script OS 6_v1 (Autodesk Fusion 360 design; units mm, degrees)
Autodesk Fusion 360 part; units mm, degrees
(part 1 of 3)
sketch "right content" plane through (0, 0, 0) normal (0, 0, 1) x (1, 0, 0)
  line L0 (-306, -8) -> (-256, -8) construction
  line L1 (-256, -128) -> (-306, -128) construction
  line L2 (-256, -8) -> (-256, -128) construction
  line L3 (-306, -128) -> (-306, -8) construction
  circle A0 centre (-298, -98) radius 1.005 construction
  point P0 (-294, -98)
  point P1 (-290, -98)
  point P2 (-298, -94)
  point P3 (-294, -94)
  point P4 (-290, -94)
  point P5 (-298, -90)
  point P6 (-294, -90)
  point P7 (-290, -90)
  point P8 (-298, -86)
  point P9 (-294, -86)
  point P10 (-290, -86)
  point P11 (-298, -82)
  point P12 (-294, -82)
  point P13 (-290, -82)
  point P14 (-298, -78)
  point P15 (-294, -78)
  point P16 (-290, -78)
  point P17 (-298, -74)
  point P18 (-294, -74)
  point P19 (-290, -74)
  point P20 (-298, -70)
  point P21 (-294, -70)
  point P22 (-290, -70)
  point P23 (-298, -66)
  point P24 (-294, -66)
  point P25 (-290, -66)
  point P26 (-298, -62)
  point P27 (-294, -62)
  point P28 (-290, -62)
  dimension "d85" = 50
  dimension "d390" = 120
  dimension "d391" = 2.01
  dimension "d394" = 4
  dimension "d395" = 4
  dimension "d403" = 30
  dimension "d404" = 8
  constraint horizontal L1
  constraint horizontal L0
  constraint vertical L2
  constraint vertical L3
  constraint coincident L1.end L3.start
  constraint coincident L0.end L2.start
  measures "d85" distance of L0.start L0.end
  measures "d390" distance of L0 L1
  measures "d391" diameter of A0
  measures "d403" distance of L1 A0.centre
  measures "d404" distance of L3 A0.centre
sketch "top content" plane through (0, 0, 0) normal (0, 0, 1) x (1, 0, 0)
  circle A0 centre (75, 95) radius 6.5
  circle A1 centre (20, 25) radius 6.5
  circle A2 centre (90.5, 79.5) radius 1.588
  circle A3 centre (59.5, 79.5) radius 1.588
  circle A4 centre (90.5, 110.5) radius 1.588
  circle A5 centre (59.5, 110.5) radius 1.588
  circle A6 centre (130, 25) radius 6.5
  line L0 (0, 0) -> (0, 120) construction
  line L1 (0, 120) -> (150, 120) construction
  line L2 (150, 120) -> (150, 0) construction
  line L3 (150, 0) -> (0, 0) construction
  line L4 (0, 0) -> (150, 120) construction
  line L5 (0, 120) -> (150, 0) construction
  line L6 (75, 0) -> (75, 120) construction
  point P0 (75, 60)
  dimension "d263" = 31
  dimension "d25" = 31
  dimension "d3" = 13
  dimension "d4" = 110
  dimension "d272" = 3.176
  dimension "d1371" = 120
  dimension "d1372" = 150
  dimension "d1373" = 25
  dimension "d1374" = 25
  dimension "d2151" = 15.5
  dimension "d2152" = 15.5
  dimension "d2153" = 55
  dimension "d2154" = 35
  constraint equal A0 A1
  constraint equal A1 A6
  constraint perpendicular L0 L1
  constraint parallel L0 L2
  constraint parallel L1 L3
  constraint coincident L4 P0
  constraint coincident L5 P0
  constraint midpoint L3 L6.start
  constraint midpoint L1 L6.end
  constraint coincident A0.centre L6
  constraint horizontal L3
  measures "d3" diameter of A1
  measures "d4" distance of A6.centre A1.centre
  measures "d272" diameter of A3
  measures "d1371" distance of L1.end L2.end
  measures "d1372" distance of L0.end L1.end
  measures "d1373" distance of A0.centre L1
  measures "d1374" distance of A6.centre L3
  measures "d2151" horizontal distance of A0.centre A2.centre
  measures "d2152" vertical distance of A0.centre A4.centre
  measures "d2153" horizontal distance of A1.centre P0
  measures "d2154" vertical distance of A1.centre P0
sketch "bottom content" plane through (0, 0, 0) normal (0, 0, 1) x (1, 0, 0)
  circle A0 centre (245.4709, 45.6033) radius 1
  circle A1 centre (385.4709, 45.6033) radius 1
  circle A2 centre (245.4709, -54.3967) radius 1
  circle A3 centre (385.4709, -54.3967) radius 1
  circle A4 centre (255.4709, 35.6033) radius 1
  circle A5 centre (375.4709, 35.6033) radius 1
  circle A6 centre (255.4709, -44.3967) radius 1
  circle A7 centre (375.4709, -44.3967) radius 1
  line L0 (235.4709, 55.6033) -> (395.4709, 55.6033) construction
  line L1 (395.4709, 55.6033) -> (395.4709, -64.3967) construction
  line L2 (395.4709, -64.3967) -> (235.4709, -64.3967) construction
  line L3 (235.4709, -64.3967) -> (235.4709, 55.6033) construction
  line L4 (235.4709, 55.6033) -> (395.4709, -64.3967) construction
  line L5 (395.4709, 55.6033) -> (235.4709, -64.3967) construction
  line L6 (268.4709, -6.3967) -> (362.4709, -6.3967) construction
  line L7 (362.4709, -6.3967) -> (362.4709, -54.3967) construction
  line L8 (362.4709, -54.3967) -> (268.4709, -54.3967) construction
  line L9 (268.4709, -54.3967) -> (268.4709, -6.3967) construction
  line L10 (315.4709, -4.3967) -> (315.4709, -64.3967) construction
  circle A8 centre (268.4709, -6.3967) radius 1
  circle A9 centre (362.4709, -6.3967) radius 1
  circle A10 centre (362.4709, -54.3967) radius 1
  circle A11 centre (268.4709, -54.3967) radius 1
  point P0 (315.4709, -4.3967)
  point P1 (315.4709, -4.3967)
  dimension "d282" = 2
  dimension "d287" = 140
  dimension "d288" = -100
  dimension "d289" = 2
  dimension "d294" = 120
  dimension "d295" = -80
  dimension "d356" = 160
  dimension "d357" = 120
  dimension "d358" = 70
  dimension "d359" = 50
  dimension "d360" = 60
  dimension "d361" = 40
  dimension "d362" = 94
  dimension "d363" = 48
  dimension "d364" = 10
  dimension "d365" = 47
  dimension "d366" = 2
  dimension "d368" = 2
  dimension "d369" = 2
  dimension "d370" = 2
  constraint horizontal L0
  constraint perpendicular L0 L1
  constraint parallel L0 L2
  constraint parallel L1 L3
  constraint coincident L4 P1
  constraint coincident L5 P1
  constraint coincident P1 P0
  constraint horizontal L6
  constraint vertical L7
  constraint horizontal L8
  constraint vertical L9
  constraint midpoint L2 L10.end
  constraint coincident L6.start L9.end
  constraint coincident L6.end L7.start
  constraint coincident L7.end L8.start
  constraint coincident L8.end L9.start
  measures "d282" diameter of A0
  measures "d289" diameter of A4
  measures "d356" distance of L1.end L2.end
  measures "d357" distance of L0.start L2.end
  measures "d358" horizontal distance of A0.centre P0
  measures "d359" vertical distance of A0.centre P0
  measures "d360" horizontal distance of A4.centre P1
  measures "d361" vertical distance of A4.centre P1
  measures "d362" distance of L6.start L6.end
  measures "d363" distance of L6.start L8.end
  measures "d364" distance of L2 L8
  measures "d365" distance of L8.end L10
  measures "d366" diameter of A8
  measures "d368" diameter of A11
  measures "d369" diameter of A9
  measures "d370" diameter of A10
sketch "back content" plane through (0, 0, 0) normal (0, 0, 1) x (1, 0, 0)
  line L0 (16.9082, 180.3872) -> (176.9082, 180.3872) construction
  line L1 (176.9082, 180.3872) -> (176.9082, 130.3872) construction
  line L2 (176.9082, 130.3872) -> (16.9082, 130.3872) construction
  line L3 (16.9082, 130.3872) -> (16.9082, 180.3872) construction
  circle A0 centre (156.9082, 150.3872) radius 5.6
  dimension "d381" = 160
  dimension "d382" = 50
  dimension "d387" = 11.2
  dimension "d388" = 20
  dimension "d389" = 20
  constraint horizontal L0
  constraint horizontal L2
  constraint vertical L3
  constraint vertical L1
  measures "d381" distance of L0.start L0.end
  measures "d382" distance of L0.start L2.end
  measures "d387" diameter of A0
  measures "d388" distance of L2 A0.centre
  measures "d389" distance of L1 A0.centre
sketch "front content" plane through (0, 0, 0) normal (0, 0, 1) x (1, 0, 0)
  line L0 (-253.343, 200.8306) -> (-230.343, 200.8306)
  line L1 (-230.343, 200.8306) -> (-230.343, 190.3306)
  line L2 (-230.343, 190.3306) -> (-253.343, 190.3306)
  line L3 (-253.343, 190.3306) -> (-253.343, 200.8306)
  circle A0 centre (-183.343, 190.8306) radius 3.5
  line L4 (-143.343, 185.8306) -> (-128.343, 185.8306)
  line L5 (-128.343, 185.8306) -> (-128.343, 177.8306)
  line L6 (-128.343, 177.8306) -> (-143.343, 177.8306)
  line L7 (-143.343, 177.8306) -> (-143.343, 185.8306)
  line L8 (-273.343, 215.8306) -> (-113.343, 215.8306) construction
  line L9 (-113.343, 215.8306) -> (-113.343, 165.8306) construction
  line L10 (-113.343, 165.8306) -> (-273.343, 165.8306) construction
  line L11 (-273.343, 165.8306) -> (-273.343, 215.8306) construction
  dimension "d332" = 23
  dimension "d333" = 10.5
  dimension "d336" = 7
  dimension "d339" = 15
  dimension "d340" = 8
  dimension "d371" = 160
  dimension "d372" = 50
  dimension "d374" = 20
  dimension "d376" = 15
  dimension "d377" = 12
  dimension "d378" = 15
  dimension "d379" = 25
  dimension "d380" = 70
  constraint horizontal L0
  constraint vertical L1
  constraint horizontal L2
  constraint vertical L3
  constraint horizontal L4
  constraint vertical L5
  constraint horizontal L6
  constraint vertical L7
  constraint horizontal L8
  constraint vertical L9
  constraint horizontal L10
  constraint vertical L11
  measures "d332" distance of L0.start L0.end
  measures "d333" distance of L0.start L2.end
  measures "d336" diameter of A0
  measures "d339" distance of L4.start L4.end
  measures "d340" distance of L4.start L6.end
  measures "d371" distance of L8.start L8.end
  measures "d372" distance of L8.start L10.end
  measures "d374" distance of L3 L11
  measures "d376" distance of L0 L8
  measures "d377" distance of L6 L10
  measures "d378" distance of L5 L9
  measures "d379" distance of A0.centre L10
  measures "d380" distance of A0.centre L9
sketch "left content" plane through (0, 0, 0) normal (0, 0, 1) x (1, 0, 0)
  line L0 (131.529, -3.2484) -> (131.529, 116.7516) construction
  circle A0 centre (139.529, 26.7516) radius 1.005 construction
  line L1 (181.529, -3.2484) -> (131.529, -3.2484) construction
  line L2 (131.529, 116.7516) -> (181.529, 116.7516) construction
  line L3 (181.529, 116.7516) -> (181.529, -3.2484) construction
  point P0 (139.529, 34.7516)
  point P1 (147.529, 50.7516)
  point P2 (139.529, 54.7516)
  point P3 (143.529, 54.7516)
  point P4 (147.529, 34.7516)
  point P5 (139.529, 30.7516)
  point P6 (143.529, 30.7516)
  point P7 (143.529, 50.7516)
  point P8 (143.529, 34.7516)
  point P9 (139.529, 38.7516)
  point P10 (147.529, 38.7516)
  point P11 (139.529, 42.7516)
  point P12 (143.529, 38.7516)
  point P13 (139.529, 46.7516)
  point P14 (147.529, 42.7516)
  point P15 (143.529, 46.7516)
  point P16 (147.529, 46.7516)
  point P17 (139.529, 50.7516)
  point P18 (143.529, 42.7516)
  point P19 (147.529, 30.7516)
  point P20 (147.529, 26.7516)
  point P21 (143.529, 26.7516)
  point P22 (143.529, 58.7516)
  point P23 (143.529, 62.7516)
  point P24 (147.529, 54.7516)
  point P25 (139.529, 58.7516)
  point P26 (147.529, 58.7516)
  point P27 (139.529, 62.7516)
  point P28 (147.529, 62.7516)
  dimension "d398" = 4
  dimension "d399" = 4
  dimension "d400" = 50
  dimension "d401" = 120
  dimension "d402" = 2.01
  dimension "d405" = 30
  dimension "d406" = 8
  constraint horizontal L1
  constraint horizontal L2
  constraint vertical L3
  constraint vertical L0
  constraint coincident L0.start L1.end
  constraint coincident L2.end L3.start
  measures "d400" distance of L2.end L0.end
  measures "d401" distance of L1 L2
  measures "d402" diameter of A0
  measures "d405" distance of A0.centre L1
  measures "d406" distance of A0.centre L0
sketch "b  stock" plane through (0, 0, 0) normal (0, 0, 1) x (1, 0, 0)
  line L0 (0, 0) -> (304.8, 0)
  line L1 (304.8, 0) -> (304.8, 609.6)
  line L2 (304.8, 609.6) -> (0, 609.6)
  line L3 (0, 609.6) -> (0, 0)
extrude "b  stock body extrude" add sketch "b  stock" along normal blind 3.175 makes body 1
sketch "b  layout" plane through (0, 0, 0) normal (0, 0, 1) x (1, 0, 0)
  line L0 (0, 0) -> (150, 0)
  line L1 (150, 0) -> (150, 120)
  line L2 (150, 120) -> (0, 120)
  line L3 (0, 120) -> (0, 0)
  line L4 (152.01, 0) -> (302.01, 0)
  line L5 (302.01, 0) -> (302.01, 120)
  line L6 (302.01, 120) -> (152.01, 120)
  line L7 (152.01, 120) -> (152.01, 0)
  line L8 (0, 122.01) -> (50, 122.01)
  line L9 (50, 122.01) -> (50, 272.01)
  line L10 (50, 272.01) -> (0, 272.01)
  line L11 (0, 272.01) -> (0, 122.01)
  line L12 (52.01, 122.01) -> (102.01, 122.01)
  line L13 (102.01, 122.01) -> (102.01, 272.01)
  line L14 (102.01, 272.01) -> (52.01, 272.01)
  line L15 (52.01, 272.01) -> (52.01, 122.01)
  line L16 (104.02, 122.01) -> (154.02, 122.01)
  line L17 (154.02, 122.01) -> (154.02, 242.01)
  line L18 (154.02, 242.01) -> (104.02, 242.01)
  line L19 (104.02, 242.01) -> (104.02, 122.01)
  line L20 (156.03, 122.01) -> (206.03, 122.01)
  line L21 (206.03, 122.01) -> (206.03, 242.01)
  line L22 (206.03, 242.01) -> (156.03, 242.01)
  line L23 (156.03, 242.01) -> (156.03, 122.01)
sketch "b top lines" plane through (0, 0, 0) normal (0, 0, 1) x (1, 0, 0) in component "b top component"
  line L0 (0, 0) -> (10.1, 0)
  line L1 (10.1, 0) -> (10.1, 3.175)
  line L2 (10.1, 3.175) -> (19.9, 3.175)
  line L3 (19.9, 3.175) -> (19.9, 0)
  line L4 (19.9, 0) -> (30.1, 0)
  line L5 (30.1, 0) -> (30.1, 3.175)
  line L6 (30.1, 3.175) -> (39.9, 3.175)
  line L7 (39.9, 3.175) -> (39.9, 0)
  line L8 (39.9, 0) -> (50.1, 0)
  line L9 (50.1, 0) -> (50.1, 3.175)
  line L10 (50.1, 3.175) -> (59.9, 3.175)
  line L11 (59.9, 3.175) -> (59.9, 0)
  line L12 (59.9, 0) -> (70.1, 0)
  line L13 (70.1, 0) -> (70.1, 3.175)
  line L14 (70.1, 3.175) -> (79.9, 3.175)
  line L15 (79.9, 3.175) -> (79.9, 0)
  line L16 (79.9, 0) -> (90.1, 0)
  line L17 (90.1, 0) -> (90.1, 3.175)
  line L18 (90.1, 3.175) -> (99.9, 3.175)
  line L19 (99.9, 3.175) -> (99.9, 0)
  line L20 (99.9, 0) -> (110.1, 0)
  line L21 (110.1, 0) -> (110.1, 3.175)
  line L22 (110.1, 3.175) -> (119.9, 3.175)
  line L23 (119.9, 3.175) -> (119.9, 0)
  line L24 (119.9, 0) -> (130.1, 0)
  line L25 (130.1, 0) -> (130.1, 3.175)
  line L26 (130.1, 3.175) -> (139.9, 3.175)
  line L27 (139.9, 3.175) -> (139.9, 0)
  line L28 (139.9, 0) -> (150, 0)
  line L29 (150, 0) -> (150, 15.1)
  line L30 (150, 15.1) -> (146.825, 15.1)
  line L31 (146.825, 15.1) -> (146.825, 24.9)
  line L32 (146.825, 24.9) -> (150, 24.9)
  line L33 (150, 24.9) -> (150, 35.1)
  line L34 (150, 35.1) -> (146.825, 35.1)
  line L35 (146.825, 35.1) -> (146.825, 44.9)
  line L36 (146.825, 44.9) -> (150, 44.9)
  line L37 (150, 44.9) -> (150, 55.1)
  line L38 (150, 55.1) -> (146.825, 55.1)
  line L39 (146.825, 55.1) -> (146.825, 64.9)
  line L40 (146.825, 64.9) -> (150, 64.9)
  line L41 (150, 64.9) -> (150, 75.1)
  line L42 (150, 75.1) -> (146.825, 75.1)
  line L43 (146.825, 75.1) -> (146.825, 84.9)
  line L44 (146.825, 84.9) -> (150, 84.9)
  line L45 (150, 84.9) -> (150, 95.1)
  line L46 (150, 95.1) -> (146.825, 95.1)
  line L47 (146.825, 95.1) -> (146.825, 104.9)
  line L48 (146.825, 104.9) -> (150, 104.9)
  line L49 (150, 104.9) -> (150, 120)
  line L50 (0, 120) -> (10.1, 120)
  line L51 (10.1, 120) -> (10.1, 116.825)
  line L52 (10.1, 116.825) -> (19.9, 116.825)
  line L53 (19.9, 116.825) -> (19.9, 120)
  line L54 (19.9, 120) -> (30.1, 120)
  line L55 (30.1, 120) -> (30.1, 116.825)
  line L56 (30.1, 116.825) -> (39.9, 116.825)
  line L57 (39.9, 116.825) -> (39.9, 120)
  line L58 (39.9, 120) -> (50.1, 120)
  line L59 (50.1, 120) -> (50.1, 116.825)
  line L60 (50.1, 116.825) -> (59.9, 116.825)
  line L61 (59.9, 116.825) -> (59.9, 120)
  line L62 (59.9, 120) -> (70.1, 120)
  line L63 (70.1, 120) -> (70.1, 116.825)
  line L64 (70.1, 116.825) -> (79.9, 116.825)
  line L65 (79.9, 116.825) -> (79.9, 120)
  line L66 (79.9, 120) -> (90.1, 120)
  line L67 (90.1, 120) -> (90.1, 116.825)
  line L68 (90.1, 116.825) -> (99.9, 116.825)
  line L69 (99.9, 116.825) -> (99.9, 120)
  line L70 (99.9, 120) -> (110.1, 120)
  line L71 (110.1, 120) -> (110.1, 116.825)
  line L72 (110.1, 116.825) -> (119.9, 116.825)
  line L73 (119.9, 116.825) -> (119.9, 120)
  line L74 (119.9, 120) -> (130.1, 120)
  line L75 (130.1, 120) -> (130.1, 116.825)
  line L76 (130.1, 116.825) -> (139.9, 116.825)
  line L77 (139.9, 116.825) -> (139.9, 120)
  line L78 (139.9, 120) -> (150, 120)
  line L79 (0, 0) -> (0, 15.1)
  line L80 (0, 15.1) -> (3.175, 15.1)
  line L81 (3.175, 15.1) -> (3.175, 24.9)
  line L82 (3.175, 24.9) -> (0, 24.9)
  line L83 (0, 24.9) -> (0, 35.1)
  line L84 (0, 35.1) -> (3.175, 35.1)
  line L85 (3.175, 35.1) -> (3.175, 44.9)
  line L86 (3.175, 44.9) -> (0, 44.9)
  line L87 (0, 44.9) -> (0, 55.1)
  line L88 (0, 55.1) -> (3.175, 55.1)
  line L89 (3.175, 55.1) -> (3.175, 64.9)
  line L90 (3.175, 64.9) -> (0, 64.9)
  line L91 (0, 64.9) -> (0, 75.1)
  line L92 (0, 75.1) -> (3.175, 75.1)
  line L93 (3.175, 75.1) -> (3.175, 84.9)
  line L94 (3.175, 84.9) -> (0, 84.9)
  line L95 (0, 84.9) -> (0, 95.1)
  line L96 (0, 95.1) -> (3.175, 95.1)
  line L97 (3.175, 95.1) -> (3.175, 104.9)
  line L98 (3.175, 104.9) -> (0, 104.9)
  line L99 (0, 104.9) -> (0, 120)
  dimension "d1431" = 10.1
  dimension "d1432" = 3.175
  dimension "d1433" = 9.8
  dimension "d1434" = 3.175
  dimension "d1435" = 10.2
  dimension "d1436" = 3.175
  dimension "d1437" = 9.8
  dimension "d1438" = 3.175
  dimension "d1439" = 10.2
  dimension "d1440" = 3.175
  dimension "d1441" = 9.8
  dimension "d1442" = 3.175
  dimension "d1443" = 10.2
  dimension "d1444" = 3.175
  dimension "d1445" = 9.8
  dimension "d1446" = 3.175
  dimension "d1447" = 10.2
  dimension "d1448" = 3.175
  dimension "d1449" = 9.8
  dimension "d1450" = 3.175
  dimension "d1451" = 10.2
  dimension "d1452" = 3.175
  dimension "d1453" = 9.8
  dimension "d1454" = 3.175
  dimension "d1455" = 10.2
  dimension "d1456" = 3.175
  dimension "d1457" = 9.8
  dimension "d1458" = 3.175
  dimension "d1459" = 10.1
  dimension "d1474" = 15.1
  dimension "d1475" = 3.175
  dimension "d1476" = 9.8
  dimension "d1477" = 3.175
  dimension "d1478" = 10.2
  dimension "d1479" = 3.175
  dimension "d1480" = 9.8
  dimension "d1481" = 3.175
  dimension "d1482" = 10.2
  dimension "d1483" = 3.175
  dimension "d1484" = 9.8
  dimension "d1485" = 3.175
  dimension "d1486" = 10.2
  dimension "d1487" = 3.175
  dimension "d1488" = 9.8
  dimension "d1489" = 3.175
  dimension "d1490" = 10.2
  dimension "d1491" = 3.175
  dimension "d1492" = 9.8
  dimension "d1493" = 3.175
  dimension "d1494" = 15.1
  dimension "d1505" = 10.1
  dimension "d1506" = 3.175
  dimension "d1507" = 9.8
  dimension "d1508" = 3.175
  dimension "d1509" = 10.2
  dimension "d1510" = 3.175
  dimension "d1511" = 9.8
  dimension "d1512" = 3.175
  dimension "d1513" = 10.2
  dimension "d1514" = 3.175
  dimension "d1515" = 9.8
  dimension "d1516" = 3.175
  dimension "d1517" = 10.2
  dimension "d1518" = 3.175
  dimension "d1519" = 9.8
  dimension "d1520" = 3.175
  dimension "d1521" = 10.2
  dimension "d1522" = 3.175
  dimension "d1523" = 9.8
  dimension "d1524" = 3.175
  dimension "d1525" = 10.2
  dimension "d1526" = 3.175
  dimension "d1527" = 9.8
  dimension "d1528" = 3.175
  dimension "d1529" = 10.2
  dimension "d1530" = 3.175
  dimension "d1531" = 9.8
  dimension "d1532" = 3.175
  dimension "d1533" = 10.1
  dimension "d1548" = 15.1
  dimension "d1549" = 3.175
  dimension "d1550" = 9.8
  dimension "d1551" = 3.175
  dimension "d1552" = 10.2
  dimension "d1553" = 3.175
  dimension "d1554" = 9.8
  dimension "d1555" = 3.175
  dimension "d1556" = 10.2
  dimension "d1557" = 3.175
  dimension "d1558" = 9.8
  dimension "d1559" = 3.175
  dimension "d1560" = 10.2
  dimension "d1561" = 3.175
  dimension "d1562" = 9.8
  dimension "d1563" = 3.175
  dimension "d1564" = 10.2
  dimension "d1565" = 3.175
  dimension "d1566" = 9.8
  dimension "d1567" = 3.175
  dimension "d1568" = 15.1
  constraint horizontal L0
  constraint vertical L1
  constraint horizontal L2
  constraint vertical L3
  constraint horizontal L4
  constraint vertical L5
  constraint horizontal L6
  constraint vertical L7
  constraint horizontal L8
  constraint vertical L9
  constraint horizontal L10
  constraint vertical L11
  constraint horizontal L12
  constraint vertical L13
  constraint horizontal L14
  constraint vertical L15
  constraint horizontal L16
  constraint vertical L17
  constraint horizontal L18
  constraint vertical L19
  constraint horizontal L20
  constraint vertical L21
  constraint horizontal L22
  constraint vertical L23
  constraint horizontal L24
  constraint vertical L25
  constraint horizontal L26
  constraint vertical L27
  constraint horizontal L28
  constraint vertical L29
  constraint horizontal L30
  constraint vertical L31
  constraint horizontal L32
  constraint vertical L33
  constraint horizontal L34
  constraint vertical L35
  constraint horizontal L36
  constraint vertical L37
  constraint horizontal L38
  constraint vertical L39
  constraint horizontal L40
  constraint vertical L41
  constraint horizontal L42
  constraint vertical L43
  constraint horizontal L44
  constraint vertical L45
  constraint horizontal L46
  constraint vertical L47
  constraint horizontal L48
  constraint vertical L49
  constraint horizontal L50
  constraint vertical L51
  constraint horizontal L52
  constraint vertical L53
  constraint horizontal L54
  constraint vertical L55
  constraint horizontal L56
  constraint vertical L57
  constraint horizontal L58
  constraint vertical L59
  constraint horizontal L60
  constraint vertical L61
  constraint horizontal L62
  constraint vertical L63
  constraint horizontal L64
  constraint vertical L65
  constraint horizontal L66
  constraint vertical L67
  constraint horizontal L68
  constraint vertical L69
  constraint horizontal L70
  constraint vertical L71
  constraint horizontal L72
  constraint vertical L73
  constraint horizontal L74
  constraint vertical L75
  constraint horizontal L76
  constraint vertical L77
  constraint horizontal L78
  constraint vertical L79
  constraint horizontal L80
  constraint vertical L81
  constraint horizontal L82
  constraint vertical L83
  constraint horizontal L84
  constraint vertical L85
  constraint horizontal L86
  constraint vertical L87
  constraint horizontal L88
  constraint vertical L89
  constraint horizontal L90
  constraint vertical L91
  constraint horizontal L92
  constraint vertical L93
  constraint horizontal L94
  constraint vertical L95
  constraint horizontal L96
  constraint vertical L97
  constraint horizontal L98
  constraint vertical L99
  measures "d1431" distance of L0.start L0.end
  measures "d1432" distance of L0.end L1.end
  measures "d1433" distance of L1.end L2.end
  measures "d1434" distance of L2.end L3.end
  measures "d1435" distance of L3.end L4.end
  measures "d1436" distance of L4.end L5.end
  measures "d1437" distance of L5.end L6.end
  measures "d1438" distance of L6.end L7.end
  measures "d1439" distance of L7.end L8.end
  measures "d1440" distance of L8.end L9.end
  measures "d1441" distance of L9.end L10.end
  measures "d1442" distance of L10.end L11.end
  measures "d1443" distance of L11.end L12.end
  measures "d1444" distance of L12.end L13.end
  measures "d1445" distance of L13.end L14.end
  measures "d1446" distance of L14.end L15.end
  measures "d1447" distance of L15.end L16.end
  measures "d1448" distance of L16.end L17.end
  measures "d1449" distance of L17.end L18.end
  measures "d1450" distance of L18.end L19.end
  measures "d1451" distance of L19.end L20.end
  measures "d1452" distance of L20.end L21.end
  measures "d1453" distance of L21.end L22.end
  measures "d1454" distance of L22.end L23.end
  measures "d1455" distance of L23.end L24.end
  measures "d1456" distance of L24.end L25.end
  measures "d1457" distance of L25.end L26.end
  measures "d1458" distance of L26.end L27.end
  measures "d1459" distance of L27.end L28.end
  measures "d1474" distance of L28.end L29.end
  measures "d1475" distance of L29.end L30.end
  measures "d1476" distance of L30.end L31.end
  measures "d1477" distance of L31.end L32.end
  measures "d1478" distance of L32.end L33.end
  measures "d1479" distance of L33.end L34.end
  measures "d1480" distance of L34.end L35.end
  measures "d1481" distance of L35.end L36.end
  measures "d1482" distance of L36.end L37.end
  measures "d1483" distance of L37.end L38.end
  measures "d1484" distance of L38.end L39.end
  measures "d1485" distance of L39.end L40.end
  measures "d1486" distance of L40.end L41.end
  measures "d1487" distance of L41.end L42.end
  measures "d1488" distance of L42.end L43.end
  measures "d1489" distance of L43.end L44.end
  measures "d1490" distance of L44.end L45.end
  measures "d1491" distance of L45.end L46.end
  measures "d1492" distance of L46.end L47.end
  measures "d1493" distance of L47.end L48.end
  measures "d1494" distance of L48.end L49.end
  measures "d1505" distance of L50.start L50.end
  measures "d1506" distance of L50.end L51.end
  measures "d1507" distance of L51.end L52.end
  measures "d1508" distance of L52.end L53.end
  measures "d1509" distance of L53.end L54.end
  measures "d1510" distance of L54.end L55.end
  measures "d1511" distance of L55.end L56.end
  measures "d1512" distance of L56.end L57.end
  measures "d1513" distance of L57.end L58.end
  measures "d1514" distance of L58.end L59.end
  measures "d1515" distance of L59.end L60.end
  measures "d1516" distance of L60.end L61.end
  measures "d1517" distance of L61.end L62.end
  measures "d1518" distance of L62.end L63.end
  measures "d1519" distance of L63.end L64.end
  measures "d1520" distance of L64.end L65.end
  measures "d1521" distance of L65.end L66.end
  measures "d1522" distance of L66.end L67.end
  measures "d1523" distance of L67.end L68.end
  measures "d1524" distance of L68.end L69.end
  measures "d1525" distance of L69.end L70.end
  measures "d1526" distance of L70.end L71.end
  measures "d1527" distance of L71.end L72.end
  measures "d1528" distance of L72.end L73.end
  measures "d1529" distance of L73.end L74.end
  measures "d1530" distance of L74.end L75.end
  measures "d1531" distance of L75.end L76.end
  measures "d1532" distance of L76.end L77.end
  measures "d1533" distance of L49.end L77.end
  measures "d1548" distance of L0.start L79.end
  measures "d1549" distance of L79.end L80.end
  measures "d1550" distance of L80.end L81.end
  measures "d1551" distance of L81.end L82.end
  measures "d1552" distance of L82.end L83.end
  measures "d1553" distance of L83.end L84.end
  measures "d1554" distance of L84.end L85.end
  measures "d1555" distance of L85.end L86.end
  measures "d1556" distance of L86.end L87.end
  measures "d1557" distance of L87.end L88.end
  measures "d1558" distance of L88.end L89.end
  measures "d1559" distance of L89.end L90.end
  measures "d1560" distance of L90.end L91.end
  measures "d1561" distance of L91.end L92.end
  measures "d1562" distance of L92.end L93.end
  measures "d1563" distance of L93.end L94.end
  measures "d1564" distance of L94.end L95.end
  measures "d1565" distance of L95.end L96.end
  measures "d1566" distance of L96.end L97.end
  measures "d1567" distance of L97.end L98.end
  measures "d1568" distance of L50.start L98.end
sketch "b top circles" plane through (0, 0, 0) normal (0, 0, 1) x (1, 0, 0) in component "b top component"
  line L0 (0, 0) -> (150, 0)
  line L1 (150, 0) -> (150, 120)
  line L2 (150, 120) -> (0, 120)
  line L3 (0, 120) -> (0, 0)
  circle A0 centre (10.6906, 2.3644) radius 1.005
  circle A1 centre (19.3094, 2.3644) radius 1.005
  circle A2 centre (30.6906, 2.3644) radius 1.005
  circle A3 centre (39.3094, 2.3644) radius 1.005
  circle A4 centre (50.6906, 2.3644) radius 1.005
  circle A5 centre (59.3094, 2.3644) radius 1.005
  circle A6 centre (70.6906, 2.3644) radius 1.005
  circle A7 centre (79.3094, 2.3644) radius 1.005
  circle A8 centre (90.6906, 2.3644) radius 1.005
  circle A9 centre (99.3094, 2.3644) radius 1.005
  circle A10 centre (110.6906, 2.3644) radius 1.005
  circle A11 centre (119.3094, 2.3644) radius 1.005
  circle A12 centre (130.6906, 2.3644) radius 1.005
  circle A13 centre (139.3094, 2.3644) radius 1.005
  circle A14 centre (147.6356, 15.6906) radius 1.005
  circle A15 centre (147.6356, 24.3094) radius 1.005
  circle A16 centre (147.6356, 35.6906) radius 1.005
  circle A17 centre (147.6356, 44.3094) radius 1.005
  circle A18 centre (147.6356, 55.6906) radius 1.005
  circle A19 centre (147.6356, 64.3094) radius 1.005
  circle A20 centre (147.6356, 75.6906) radius 1.005
  circle A21 centre (147.6356, 84.3094) radius 1.005
  circle A22 centre (147.6356, 95.6906) radius 1.005
  circle A23 centre (147.6356, 104.3094) radius 1.005
  circle A24 centre (10.6906, 117.6356) radius 1.005
  circle A25 centre (19.3094, 117.6356) radius 1.005
  circle A26 centre (30.6906, 117.6356) radius 1.005
  circle A27 centre (39.3094, 117.6356) radius 1.005
  circle A28 centre (50.6906, 117.6356) radius 1.005
  circle A29 centre (59.3094, 117.6356) radius 1.005
  circle A30 centre (70.6906, 117.6356) radius 1.005
  circle A31 centre (79.3094, 117.6356) radius 1.005
  circle A32 centre (90.6906, 117.6356) radius 1.005
  circle A33 centre (99.3094, 117.6356) radius 1.005
  circle A34 centre (110.6906, 117.6356) radius 1.005
  circle A35 centre (119.3094, 117.6356) radius 1.005
  circle A36 centre (130.6906, 117.6356) radius 1.005
  circle A37 centre (139.3094, 117.6356) radius 1.005
  circle A38 centre (2.3644, 15.6906) radius 1.005
  circle A39 centre (2.3644, 24.3094) radius 1.005
  circle A40 centre (2.3644, 35.6906) radius 1.005
  circle A41 centre (2.3644, 44.3094) radius 1.005
  circle A42 centre (2.3644, 55.6906) radius 1.005
  circle A43 centre (2.3644, 64.3094) radius 1.005
  circle A44 centre (2.3644, 75.6906) radius 1.005
  circle A45 centre (2.3644, 84.3094) radius 1.005
  circle A46 centre (2.3644, 95.6906) radius 1.005
  circle A47 centre (2.3644, 104.3094) radius 1.005
  dimension "d1460" = 2.01
  dimension "d1461" = 2.01
  dimension "d1462" = 2.01
  dimension "d1463" = 2.01
  dimension "d1464" = 2.01
  dimension "d1465" = 2.01
  dimension "d1466" = 2.01
  dimension "d1467" = 2.01
  dimension "d1468" = 2.01
  dimension "d1469" = 2.01
  dimension "d1470" = 2.01
  dimension "d1471" = 2.01
  dimension "d1472" = 2.01
  dimension "d1473" = 2.01
  dimension "d1495" = 2.01
  dimension "d1496" = 2.01
  dimension "d1497" = 2.01
  dimension "d1498" = 2.01
  dimension "d1499" = 2.01
  dimension "d1500" = 2.01
  dimension "d1501" = 2.01
  dimension "d1502" = 2.01
  dimension "d1503" = 2.01
  dimension "d1504" = 2.01
  dimension "d1534" = 2.01
  dimension "d1535" = 2.01
  dimension "d1536" = 2.01
  dimension "d1537" = 2.01
  dimension "d1538" = 2.01
  dimension "d1539" = 2.01
  dimension "d1540" = 2.01
  dimension "d1541" = 2.01
  dimension "d1542" = 2.01
  dimension "d1543" = 2.01
  dimension "d1544" = 2.01
  dimension "d1545" = 2.01
  dimension "d1546" = 2.01
  dimension "d1547" = 2.01
  dimension "d1569" = 2.01
  dimension "d1570" = 2.01
  dimension "d1571" = 2.01
  dimension "d1572" = 2.01
  dimension "d1573" = 2.01
  dimension "d1574" = 2.01
  dimension "d1575" = 2.01
  dimension "d1576" = 2.01
  dimension "d1577" = 2.01
  dimension "d1578" = 2.01
  measures "d1460" diameter of A0
  measures "d1461" diameter of A1
  measures "d1462" diameter of A2
  measures "d1463" diameter of A3
  measures "d1464" diameter of A4
  measures "d1465" diameter of A5
  measures "d1466" diameter of A6
  measures "d1467" diameter of A7
  measures "d1468" diameter of A8
  measures "d1469" diameter of A9
  measures "d1470" diameter of A10
  measures "d1471" diameter of A11
  measures "d1472" diameter of A12
  measures "d1473" diameter of A13
  measures "d1495" diameter of A14
  measures "d1496" diameter of A15
  measures "d1497" diameter of A16
  measures "d1498" diameter of A17
  measures "d1499" diameter of A18
  measures "d1500" diameter of A19
  measures "d1501" diameter of A20
  measures "d1502" diameter of A21
  measures "d1503" diameter of A22
  measures "d1504" diameter of A23
  measures "d1534" diameter of A24
  measures "d1535" diameter of A25
  measures "d1536" diameter of A26
  measures "d1537" diameter of A27
  measures "d1538" diameter of A28
  measures "d1539" diameter of A29
  measures "d1540" diameter of A30
  measures "d1541" diameter of A31
  measures "d1542" diameter of A32
  measures "d1543" diameter of A33
  measures "d1544" diameter of A34
  measures "d1545" diameter of A35
  measures "d1546" diameter of A36
  measures "d1547" diameter of A37
  measures "d1569" diameter of A38
  measures "d1570" diameter of A39
  measures "d1571" diameter of A40
  measures "d1572" diameter of A41
  measures "d1573" diameter of A42
  measures "d1574" diameter of A43
  measures "d1575" diameter of A44
  measures "d1576" diameter of A45
  measures "d1577" diameter of A46
  measures "d1578" diameter of A47
extrude "b top lines body extrude" add sketch "b top lines" along normal blind 3.175 separate body makes body 2 in component "b top component"
extrude "b top circles extrude" add sketch "b top circles" along normal blind 3.175 separate body makes body 3 in component "b top component"
combine "b top lines final combine feature" operation intersect target body 2 tool bodies 3 in component "b top component"
sketch "b bottom lines" plane through (0, 0, 0) normal (0, 0, 1) x (1, 0, 0) in component "b bottom component"
  line L0 (152.01, 0) -> (162.11, 0)
  line L1 (162.11, 0) -> (162.11, 3.175)
  line L2 (162.11, 3.175) -> (171.91, 3.175)
  line L3 (171.91, 3.175) -> (171.91, 0)
  line L4 (171.91, 0) -> (182.11, 0)
  line L5 (182.11, 0) -> (182.11, 3.175)
  line L6 (182.11, 3.175) -> (191.91, 3.175)
  line L7 (191.91, 3.175) -> (191.91, 0)
  line L8 (191.91, 0) -> (202.11, 0)
  line L9 (202.11, 0) -> (202.11, 3.175)
  line L10 (202.11, 3.175) -> (211.91, 3.175)
  line L11 (211.91, 3.175) -> (211.91, 0)
  line L12 (211.91, 0) -> (222.11, 0)
  line L13 (222.11, 0) -> (222.11, 3.175)
  line L14 (222.11, 3.175) -> (231.91, 3.175)
  line L15 (231.91, 3.175) -> (231.91, 0)
  line L16 (231.91, 0) -> (242.11, 0)
  line L17 (242.11, 0) -> (242.11, 3.175)
  line L18 (242.11, 3.175) -> (251.91, 3.175)
  line L19 (251.91, 3.175) -> (251.91, 0)
  line L20 (251.91, 0) -> (262.11, 0)
  line L21 (262.11, 0) -> (262.11, 3.175)
  line L22 (262.11, 3.175) -> (271.91, 3.175)
  line L23 (271.91, 3.175) -> (271.91, 0)
  line L24 (271.91, 0) -> (282.11, 0)
  line L25 (282.11, 0) -> (282.11, 3.175)
  line L26 (282.11, 3.175) -> (291.91, 3.175)
  line L27 (291.91, 3.175) -> (291.91, 0)
  line L28 (291.91, 0) -> (302.01, 0)
  line L29 (302.01, 0) -> (302.01, 15.1)
  line L30 (302.01, 15.1) -> (298.835, 15.1)
  line L31 (298.835, 15.1) -> (298.835, 24.9)
  line L32 (298.835, 24.9) -> (302.01, 24.9)
  line L33 (302.01, 24.9) -> (302.01, 35.1)
  line L34 (302.01, 35.1) -> (298.835, 35.1)
  line L35 (298.835, 35.1) -> (298.835, 44.9)
  line L36 (298.835, 44.9) -> (302.01, 44.9)
  line L37 (302.01, 44.9) -> (302.01, 55.1)
  line L38 (302.01, 55.1) -> (298.835, 55.1)
  line L39 (298.835, 55.1) -> (298.835, 64.9)
  line L40 (298.835, 64.9) -> (302.01, 64.9)
  line L41 (302.01, 64.9) -> (302.01, 75.1)
  line L42 (302.01, 75.1) -> (298.835, 75.1)
  line L43 (298.835, 75.1) -> (298.835, 84.9)
  line L44 (298.835, 84.9) -> (302.01, 84.9)
  line L45 (302.01, 84.9) -> (302.01, 95.1)
  line L46 (302.01, 95.1) -> (298.835, 95.1)
  line L47 (298.835, 95.1) -> (298.835, 104.9)
  line L48 (298.835, 104.9) -> (302.01, 104.9)
  line L49 (302.01, 104.9) -> (302.01, 120)
  line L50 (152.01, 120) -> (162.11, 120)
  line L51 (162.11, 120) -> (162.11, 116.825)
  line L52 (162.11, 116.825) -> (171.91, 116.825)
  line L53 (171.91, 116.825) -> (171.91, 120)
  line L54 (171.91, 120) -> (182.11, 120)
  line L55 (182.11, 120) -> (182.11, 116.825)
  line L56 (182.11, 116.825) -> (191.91, 116.825)
  line L57 (191.91, 116.825) -> (191.91, 120)
  line L58 (191.91, 120) -> (202.11, 120)
  line L59 (202.11, 120) -> (202.11, 116.825)
  line L60 (202.11, 116.825) -> (211.91, 116.825)
  line L61 (211.91, 116.825) -> (211.91, 120)
  line L62 (211.91, 120) -> (222.11, 120)
  line L63 (222.11, 120) -> (222.11, 116.825)
  line L64 (222.11, 116.825) -> (231.91, 116.825)
  line L65 (231.91, 116.825) -> (231.91, 120)
  line L66 (231.91, 120) -> (242.11, 120)
  line L67 (242.11, 120) -> (242.11, 116.825)
  line L68 (242.11, 116.825) -> (251.91, 116.825)
  line L69 (251.91, 116.825) -> (251.91, 120)
  line L70 (251.91, 120) -> (262.11, 120)
  line L71 (262.11, 120) -> (262.11, 116.825)
  line L72 (262.11, 116.825) -> (271.91, 116.825)
  line L73 (271.91, 116.825) -> (271.91, 120)
  line L74 (271.91, 120) -> (282.11, 120)
  line L75 (282.11, 120) -> (282.11, 116.825)
  line L76 (282.11, 116.825) -> (291.91, 116.825)
  line L77 (291.91, 116.825) -> (291.91, 120)
  line L78 (291.91, 120) -> (302.01, 120)
  line L79 (152.01, 0) -> (152.01, 15.1)
  line L80 (152.01, 15.1) -> (155.185, 15.1)
  line L81 (155.185, 15.1) -> (155.185, 24.9)
  line L82 (155.185, 24.9) -> (152.01, 24.9)
  line L83 (152.01, 24.9) -> (152.01, 35.1)
  line L84 (152.01, 35.1) -> (155.185, 35.1)
  line L85 (155.185, 35.1) -> (155.185, 44.9)
  line L86 (155.185, 44.9) -> (152.01, 44.9)
  line L87 (152.01, 44.9) -> (152.01, 55.1)
  line L88 (152.01, 55.1) -> (155.185, 55.1)
  line L89 (155.185, 55.1) -> (155.185, 64.9)
  line L90 (155.185, 64.9) -> (152.01, 64.9)
  line L91 (152.01, 64.9) -> (152.01, 75.1)
  line L92 (152.01, 75.1) -> (155.185, 75.1)
  line L93 (155.185, 75.1) -> (155.185, 84.9)
  line L94 (155.185, 84.9) -> (152.01, 84.9)
  line L95 (152.01, 84.9) -> (152.01, 95.1)
  line L96 (152.01, 95.1) -> (155.185, 95.1)
  line L97 (155.185, 95.1) -> (155.185, 104.9)
  line L98 (155.185, 104.9) -> (152.01, 104.9)
  line L99 (152.01, 104.9) -> (152.01, 120)
  dimension "d1583" = 10.1
  dimension "d1584" = 3.175
  dimension "d1585" = 9.8
  dimension "d1586" = 3.175
  dimension "d1587" = 10.2
  dimension "d1588" = 3.175
  dimension "d1589" = 9.8
  dimension "d1590" = 3.175
  dimension "d1591" = 10.2
  dimension "d1592" = 3.175
  dimension "d1593" = 9.8
  dimension "d1594" = 3.175
  dimension "d1595" = 10.2
  dimension "d1596" = 3.175
  dimension "d1597" = 9.8
  dimension "d1598" = 3.175
  dimension "d1599" = 10.2
  dimension "d1600" = 3.175
  dimension "d1601" = 9.8
  dimension "d1602" = 3.175
  dimension "d1603" = 10.2
  dimension "d1604" = 3.175
  dimension "d1605" = 9.8
  dimension "d1606" = 3.175
  dimension "d1607" = 10.2
  dimension "d1608" = 3.175
  dimension "d1609" = 9.8
  dimension "d1610" = 3.175
  dimension "d1611" = 10.1
  dimension "d1626" = 15.1
  dimension "d1627" = 3.175
  dimension "d1628" = 9.8
  dimension "d1629" = 3.175
  dimension "d1630" = 10.2
  dimension "d1631" = 3.175
  dimension "d1632" = 9.8
  dimension "d1633" = 3.175
  dimension "d1634" = 10.2
  dimension "d1635" = 3.175
  dimension "d1636" = 9.8
  dimension "d1637" = 3.175
  dimension "d1638" = 10.2
  dimension "d1639" = 3.175
  dimension "d1640" = 9.8
  dimension "d1641" = 3.175
  dimension "d1642" = 10.2
  dimension "d1643" = 3.175
  dimension "d1644" = 9.8
  dimension "d1645" = 3.175
  dimension "d1646" = 15.1
  dimension "d1657" = 10.1
  dimension "d1658" = 3.175
  dimension "d1659" = 9.8
  dimension "d1660" = 3.175
  dimension "d1661" = 10.2
  dimension "d1662" = 3.175
  dimension "d1663" = 9.8
  dimension "d1664" = 3.175
  dimension "d1665" = 10.2
  dimension "d1666" = 3.175
  dimension "d1667" = 9.8
  dimension "d1668" = 3.175
  dimension "d1669" = 10.2
  dimension "d1670" = 3.175
  dimension "d1671" = 9.8
  dimension "d1672" = 3.175
  dimension "d1673" = 10.2
  dimension "d1674" = 3.175
  dimension "d1675" = 9.8
  dimension "d1676" = 3.175
  dimension "d1677" = 10.2
  dimension "d1678" = 3.175
  dimension "d1679" = 9.8
  dimension "d1680" = 3.175
  dimension "d1681" = 10.2
  dimension "d1682" = 3.175
  dimension "d1683" = 9.8
  dimension "d1684" = 3.175
  dimension "d1685" = 10.1
  dimension "d1700" = 15.1
  dimension "d1701" = 3.175
  dimension "d1702" = 9.8
  dimension "d1703" = 3.175
  dimension "d1704" = 10.2
  dimension "d1705" = 3.175
  dimension "d1706" = 9.8
  dimension "d1707" = 3.175
  dimension "d1708" = 10.2
  dimension "d1709" = 3.175
  dimension "d1710" = 9.8
  dimension "d1711" = 3.175
  dimension "d1712" = 10.2
  dimension "d1713" = 3.175
  dimension "d1714" = 9.8
  dimension "d1715" = 3.175
  dimension "d1716" = 10.2
  dimension "d1717" = 3.175
  dimension "d1718" = 9.8
  dimension "d1719" = 3.175
  dimension "d1720" = 15.1
  constraint horizontal L0
  constraint vertical L1
  constraint horizontal L2
  constraint vertical L3
  constraint horizontal L4
  constraint vertical L5
  constraint horizontal L6
  constraint vertical L7
  constraint horizontal L8
  constraint vertical L9
  constraint horizontal L10
  constraint vertical L11
  constraint horizontal L12
  constraint vertical L13
  constraint horizontal L14
  constraint vertical L15
  constraint horizontal L16
  constraint vertical L17
  constraint horizontal L18
  constraint vertical L19
  constraint horizontal L20
  constraint vertical L21
  constraint horizontal L22
  constraint vertical L23
  constraint horizontal L24
  constraint vertical L25
  constraint horizontal L26
  constraint vertical L27
  constraint horizontal L28
  constraint vertical L29
  constraint horizontal L30
  constraint vertical L31
  constraint horizontal L32
  constraint vertical L33
  constraint horizontal L34
  constraint vertical L35
  constraint horizontal L36
  constraint vertical L37
  constraint horizontal L38
  constraint vertical L39
  constraint horizontal L40
  constraint vertical L41
  constraint horizontal L42
  constraint vertical L43
  constraint horizontal L44
  constraint vertical L45
  constraint horizontal L46
  constraint vertical L47
  constraint horizontal L48
  constraint vertical L49
  constraint horizontal L50
  constraint vertical L51
  constraint horizontal L52
  constraint vertical L53
  constraint horizontal L54
  constraint vertical L55
  constraint horizontal L56
  constraint vertical L57
  constraint horizontal L58
  constraint vertical L59
  constraint horizontal L60
  constraint vertical L61
  constraint horizontal L62
  constraint vertical L63
  constraint horizontal L64
  constraint vertical L65
  constraint horizontal L66
  constraint vertical L67
  constraint horizontal L68
  constraint vertical L69
  constraint horizontal L70
  constraint vertical L71
  constraint horizontal L72
  constraint vertical L73
  constraint horizontal L74
  constraint vertical L75
  constraint horizontal L76
  constraint vertical L77
  constraint horizontal L78
  constraint vertical L79
  constraint horizontal L80
  constraint vertical L81
  constraint horizontal L82
  constraint vertical L83
  constraint horizontal L84
  constraint vertical L85
  constraint horizontal L86
  constraint vertical L87
  constraint horizontal L88
  constraint vertical L89
  constraint horizontal L90
  constraint vertical L91
  constraint horizontal L92
  constraint vertical L93
  constraint horizontal L94
  constraint vertical L95
  constraint horizontal L96
  constraint vertical L97
  constraint horizontal L98
  constraint vertical L99
  measures "d1583" distance of L0.start L0.end
  measures "d1584" distance of L0.end L1.end
  measures "d1585" distance of L1.end L2.end
  measures "d1586" distance of L2.end L3.end
  measures "d1587" distance of L3.end L4.end
  measures "d1588" distance of L4.end L5.end
  measures "d1589" distance of L5.end L6.end
  measures "d1590" distance of L6.end L7.end
  measures "d1591" distance of L7.end L8.end
  measures "d1592" distance of L8.end L9.end
  measures "d1593" distance of L9.end L10.end
  measures "d1594" distance of L10.end L11.end
  measures "d1595" distance of L11.end L12.end
  measures "d1596" distance of L12.end L13.end
  measures "d1597" distance of L13.end L14.end
  measures "d1598" distance of L14.end L15.end
  measures "d1599" distance of L15.end L16.end
  measures "d1600" distance of L16.end L17.end
  measures "d1601" distance of L17.end L18.end
  measures "d1602" distance of L18.end L19.end
  measures "d1603" distance of L19.end L20.end
  measures "d1604" distance of L20.end L21.end
  measures "d1605" distance of L21.end L22.end
  measures "d1606" distance of L22.end L23.end
  measures "d1607" distance of L23.end L24.end
  measures "d1608" distance of L24.end L25.end
  measures "d1609" distance of L25.end L26.end
  measures "d1610" distance of L26.end L27.end
  measures "d1611" distance of L27.end L28.end
  measures "d1626" distance of L28.end L29.end
  measures "d1627" distance of L29.end L30.end
  measures "d1628" distance of L30.end L31.end
  measures "d1629" distance of L31.end L32.end
  measures "d1630" distance of L32.end L33.end
  measures "d1631" distance of L33.end L34.end
  measures "d1632" distance of L34.end L35.end
  measures "d1633" distance of L35.end L36.end
  measures "d1634" distance of L36.end L37.end
  measures "d1635" distance of L37.end L38.end
  measures "d1636" distance of L38.end L39.end
  measures "d1637" distance of L39.end L40.end
  measures "d1638" distance of L40.end L41.end
  measures "d1639" distance of L41.end L42.end
  measures "d1640" distance of L42.end L43.end
  measures "d1641" distance of L43.end L44.end
  measures "d1642" distance of L44.end L45.end
  measures "d1643" distance of L45.end L46.end
  measures "d1644" distance of L46.end L47.end
  measures "d1645" distance of L47.end L48.end
  measures "d1646" distance of L48.end L49.end
  measures "d1657" distance of L50.start L50.end
  measures "d1658" distance of L50.end L51.end
  measures "d1659" distance of L51.end L52.end
  measures "d1660" distance of L52.end L53.end
  measures "d1661" distance of L53.end L54.end
  measures "d1662" distance of L54.end L55.end
  measures "d1663" distance of L55.end L56.end
  measures "d1664" distance of L56.end L57.end
  measures "d1665" distance of L57.end L58.end
  measures "d1666" distance of L58.end L59.end
  measures "d1667" distance of L59.end L60.end
  measures "d1668" distance of L60.end L61.end
  measures "d1669" distance of L61.end L62.end
  measures "d1670" distance of L62.end L63.end
  measures "d1671" distance of L63.end L64.end
  measures "d1672" distance of L64.end L65.end
  measures "d1673" distance of L65.end L66.end
  measures "d1674" distance of L66.end L67.end
  measures "d1675" distance of L67.end L68.end
  measures "d1676" distance of L68.end L69.end
  measures "d1677" distance of L69.end L70.end
  measures "d1678" distance of L70.end L71.end
  measures "d1679" distance of L71.end L72.end
  measures "d1680" distance of L72.end L73.end
  measures "d1681" distance of L73.end L74.end
  measures "d1682" distance of L74.end L75.end
  measures "d1683" distance of L75.end L76.end
  measures "d1684" distance of L76.end L77.end
  measures "d1685" distance of L49.end L77.end
  measures "d1700" distance of L0.start L79.end
  measures "d1701" distance of L79.end L80.end
  measures "d1702" distance of L80.end L81.end
  measures "d1703" distance of L81.end L82.end
  measures "d1704" distance of L82.end L83.end
  measures "d1705" distance of L83.end L84.end
  measures "d1706" distance of L84.end L85.end
  measures "d1707" distance of L85.end L86.end
  measures "d1708" distance of L86.end L87.end
  measures "d1709" distance of L87.end L88.end
  measures "d1710" distance of L88.end L89.end
  measures "d1711" distance of L89.end L90.end
  measures "d1712" distance of L90.end L91.end
  measures "d1713" distance of L91.end L92.end
  measures "d1714" distance of L92.end L93.end
  measures "d1715" distance of L93.end L94.end
  measures "d1716" distance of L94.end L95.end
  measures "d1717" distance of L95.end L96.end
  measures "d1718" distance of L96.end L97.end
  measures "d1719" distance of L97.end L98.end
  measures "d1720" distance of L50.start L98.end